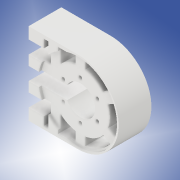
# Autodesk Inventor part: SJ001
Saved by Autodesk Inventor 2017 (Build 210142000, 142)
## iProperties
Created: 2017-06-03
Part Number: SJ001
Material: ABS Plastic
Document SubType Name: Modeling
Designer: Zach
Density: 1.06 g/cm^3
Appearance: CR White
Author: Zach
Autodesk Inventor part; units mm, degrees
ref_plane "YZ Plane" through (0, 0, 0) normal (1, 0, 0) x (0, 1, 0)
ref_plane "XZ Plane" through (0, 0, 0) normal (0, 1, 0) x (-1, 0, 0)
ref_plane "XY Plane" through (0, 0, 0) normal (0, 0, 1) x (1, 0, 0)
sketch "Sketch1" plane through (0, 0, 0) normal (0, 0, 1) x (1, 0, 0)
  circle A0 centre (0, 0) radius 62.5 construction
  line L0 (0, 62.5) -> (-75, 62.5)
  line L1 (-75, 62.5) -> (-75, -62.5)
  line L2 (-75, -62.5) -> (0, -62.5)
  arc A1 (0, -62.5) -> (0, 62.5) centre (0, 0) ccw
  dimension "d0" = 125
  dimension "d1" = 75
  dimension "d2" = 75
  constraints: 6 end point, 4 point on circle, 4 tangent, 2 centre point, 1 coincident, 1 concentric, 1 horizontal, 1 perpendicular
  measures "d0" diameter of A0
  measures "d1" distance of L0.start L0.end
  measures "d2" distance of L1.end L2.end
extrude "Extrusion1" add sketch "Sketch1" along normal blind 50
sketch "Sketch6" plane through (0, 0, 50) normal (0, 0, 1) x (1, 0, 0)
  circle A0 centre (0, 0) radius 22.5
  arc A1 (0, -62.5) -> (0, 62.5) centre (0, 0) ccw projected
  dimension "d125" = 45
  constraints: 1 centre point, 1 coincident
  measures "d125" diameter of A0
extrude "Extrusion6" cut sketch "Sketch6" against normal blind 40
sketch "Sketch7" plane through (0, 0, 50) normal (0, 0, 1) x (1, 0, 0)
  line L0 (0, 10) -> (-75, 10)
  line L1 (-75, 10) -> (-75, -10)
  line L2 (-75, -10) -> (0, -10)
  line L3 (0, -10) -> (0, 10)
  circle A0 centre (0, 0) radius 22.5 projected
  line L4 (-75, 62.5) -> (-75, -62.5) projected
  point P0 (-75, 0)
  dimension "d28" = 20
  constraints: 8 end point, 3 midpoint, 2 parallel, 1 coincident, 1 horizontal, 1 perpendicular
  measures "d28" distance of L1.end L0.end
extrude "Extrusion7" cut sketch "Sketch7" against normal blind 40 contours L3 L2 A0 L0 | A0 L2 L1 L0 picked at (-7.5, 0)
sketch "Sketch9" plane through (0, 0, 50) normal (0, 0, 1) x (1, 0, 0)
  circle A0 centre (0, 30) radius 2.5
  circle A1 centre (-25.9808, 15) radius 2.5
  circle A2 centre (-25.9808, -15) radius 2.5
  circle A3 centre (0, -30) radius 2.5
  circle A4 centre (25.9808, -15) radius 2.5
  circle A5 centre (25.9808, 15) radius 2.5
  circle A6 centre (0, 0) radius 30 construction
  dimension "d123" = 60
  dimension "d35" = 5
  dimension "d39" = 360
  constraints: 6 centre point, 2 vertical alignment, 1 coincident, 15 other
  measures "d35" diameter of A0
extrude "Extrusion9" cut sketch "Sketch9" against normal through all
sketch "Sketch10" plane through (0, 0, 50) normal (0, 0, 1) x (1, 0, 0)
  circle A0 centre (0, 0) radius 45
  arc A1 (0, -57.5) -> (0, -57.5) centre (0, 0) ccw
  line L0 (0, -57.5) -> (-75, -57.5)
  line L1 (-75, 57.5) -> (-75, -57.5)
  line L2 (0, -57.5) -> (-75, -57.5)
  line L3 (0, 57.5) -> (-75, 57.5)
  circle A2 centre (0, 0) radius 57.5 construction
  arc A3 (0, -57.5) -> (0, 57.5) centre (0, 0) ccw
  line L4 (-75, -10) -> (-75, 10)
  line L5 (0, 62.5) -> (-75, 62.5) construction
  point P0 (-75, 0)
  dimension "d111" = 115
  dimension "d43" = 90
  dimension "d114" = 90
  dimension "d124" = 5
  constraints: 10 end point, 4 point on circle, 3 centre point, 3 coincident, 2 midpoint, 2 tangent, 1 perpendicular, 1 vertical alignment, 3 other
  measures "d43" diameter of A0
  measures "d114" angle of L1 L3
  measures "d124" distance between parallel lines of L5 L3
extrude "Extrusion10" cut sketch "Sketch10" against normal blind 40
sketch "Sketch12" plane through (0, 0, 10) normal (0, 0, 1) x (1, 0, 0)
  line L0 (0, 0) -> (77.9423, -45) construction
  line L1 (0, 0) -> (90, 0) construction
  line L2 (42.1761, -15.6901) -> (57.4855, -24.529)
  line L3 (34.6761, -28.6805) -> (49.9855, -37.5194)
  arc A0 (34.6761, -28.6805) -> (42.1761, -15.6901) centre (-6.5739, 3.7955) ccw
  arc A1 (49.9877, -37.5164) -> (57.484, -24.5324) centre (-4.3593, 2.5168) ccw
  line L4 (34.6761, 28.6805) -> (49.9855, 37.5194)
  arc A2 (42.1761, 15.6901) -> (34.6761, 28.6805) centre (-6.5739, -3.7955) ccw
  line L5 (42.1761, 15.6901) -> (57.4855, 24.529)
  arc A3 (57.4855, 24.529) -> (49.9855, 37.5194) centre (-4.3593, -2.5168) ccw
  line L6 (0, 0) -> (0, -109.4234) construction
  line L7 (7.5, -44.3706) -> (7.5, -62.0484)
  line L8 (-7.5, -44.3706) -> (-7.5, -62.5)
  line L9 (0, -62.5) -> (-7.5, -62.5)
  arc A4 (-7.5, -44.3706) -> (7.5, -44.3706) centre (0, 0) ccw
  line L10 (-7.5, 44.3706) -> (-7.5, 62.5)
  line L11 (0, 62.5) -> (-7.5, 62.5)
  arc A5 (7.5, 44.3706) -> (-7.5, 44.3706) centre (0, 0) ccw
  arc A6 (-43.8748, -10) -> (-43.8748, 10) centre (0, 0) ccw projected
  arc A7 (0, -62.5) -> (0, 62.5) centre (0, 0) ccw projected
  line L12 (-75, -62.5) -> (0, -62.5) construction
  arc A8 (0, -62.5) -> (7.5, -62.0484) centre (0, 0) ccw
  line L13 (7.5, 44.3706) -> (7.5, 62.0484)
  arc A9 (7.5, 62.0484) -> (0, 62.5) centre (0, 0) ccw
  line L14 (-75, -62.5) -> (0, -62.5) projected
  line L15 (0, 62.5) -> (-75, 62.5) projected
  point P0 (54.0974, -31.2332)
  point P1 (31.1247, 32.5)
  point P2 (40, 20.6155)
  dimension "d50" = 30
  dimension "d52" = 15
  dimension "d53" = 52.5
  dimension "d54" = 67.5
  dimension "d57" = 60
  dimension "d61" = 15
  constraints: 26 end point, 24 point on circle, 8 centre point, 3 concentric, 3 point on line, 2 symmetric about line, 2 vertical, 1 equal length, 1 horizontal, 1 parallel, 14 other
  measures "d50" angle of L0 L1
  measures "d52" distance between parallel lines of L3 L2
  measures "d53" radius of A0
  measures "d54" radius of A1
  measures "d61" distance between parallel lines of L8 L7
extrude "Extrusion11" add sketch "Sketch12" along normal blind 40 contours A6 A0 | L2 A7 A1 L3 A6 | A6 L4 A3 L5 | A2 A6 | A7 A1 | A3 A7 | L7 A7 L9 L8 A4 | A5 L10 L11 A7 L13
sketch "Sketch16" plane through (0, 0, 10) normal (0, 0, 1) x (1, 0, 0)
  line L0 (-75, -62.5) -> (0, -62.5) projected
  line L1 (0, 62.5) -> (-75, 62.5) projected
  line L2 (-45, -62.5) -> (-30, -62.5)
  line L3 (-30, -62.5) -> (-30, -33.541)
  line L4 (-30, 33.541) -> (-30, 62.5)
  line L5 (-30, 62.5) -> (-45, 62.5)
  line L6 (-20.1556, -10) -> (-43.8748, -10) projected
  line L7 (-43.8748, 10) -> (-20.1556, 10) projected
  line L8 (-43.8748, 10) -> (-45, 10)
  line L9 (-43.8748, -10) -> (-45, -10)
  line L10 (-45, -10) -> (-45, -62.5)
  line L11 (-45, 62.5) -> (-45, 10)
  arc A0 (-7.5, 44.3706) -> (-43.8748, 10) centre (0, 0) ccw construction
  arc A1 (-43.8748, -10) -> (-7.5, -44.3706) centre (0, 0) ccw construction
  arc A2 (-43.8748, -10) -> (-30, -33.541) centre (0, 0) ccw
  arc A3 (-30, 33.541) -> (-43.8748, 10) centre (0, 0) ccw
  circle A4 centre (0, 0) radius 45 construction
  line L12 (-45, 10) -> (-45, -10) construction
  dimension "d127" = 15
  constraints: 18 end point, 7 point on line, 4 concentric, 4 point on circle, 3 centre point, 2 collinear, 2 vertical, 2 vertical alignment, 1 coincident, 1 perpendicular, 1 tangent
  measures "d127" distance of L2.start L2.end
extrude "Extrusion14" add sketch "Sketch16" along normal blind 40
sketch "Sketch17" plane through (0, 0, 10) normal (0, 0, 1) x (1, 0, 0)
  line L0 (-45, 10) -> (-75, 10)
  line L1 (-75, -57.5) -> (-75, 57.5) projected
  line L2 (-45, 25) -> (-75, 25)
  line L3 (-45, -10) -> (-75, -10)
  line L4 (-45, -25) -> (-75, -25)
  line L5 (-45, 25) -> (-45, 10)
  line L6 (-75, 25) -> (-75, 10)
  line L7 (-75, -10) -> (-75, -25)
  line L8 (-45, -10) -> (-45, -25)
  point P0 (0, 0)
  dimension "d39" = 360
  dimension "d72" = 15
  dimension "d73" = 15
  constraints: 16 end point, 3 point on line, 2 coincident, 2 collinear, 2 horizontal, 2 perpendicular
  measures "d72" distance between parallel lines of L0 L2
  measures "d73" distance between parallel lines of L4 L3
extrude "Extrusion15" add sketch "Sketch17" along normal blind 40
sketch "Sketch19" plane through (0, 0, 10) normal (0, 0, 1) x (1, 0, 0)
  line L0 (-75, 62.5) -> (-51.5388, 62.5)
  line L1 (-75, 25) -> (-75, 10) projected
  line L2 (-51.5388, 62.5) -> (-75, 62.5)
  line L3 (-75, 62.5) -> (-75, 45)
  line L4 (-75, 45) -> (-51.5388, 45)
  line L5 (-51.5388, 45) -> (-51.5388, 62.5)
  line L6 (-51.5388, -62.5) -> (-75, -62.5)
  line L7 (-75, 62.5) -> (-75, -62.5) projected
  line L8 (-51.5388, -62.5) -> (-75, -62.5)
  line L9 (-75, -62.5) -> (-75, -45)
  line L10 (-75, -45) -> (-51.5388, -45)
  line L11 (-51.5388, -45) -> (-51.5388, -62.5)
  point P0 (0, 0)
  point P1 (-75, -25)
  dimension "d84" = 17.5
  dimension "d85" = 17.5
  constraints: 20 end point, 4 parallel, 2 horizontal, 2 perpendicular, 2 point on line
  measures "d84" distance of L3.end L2.end
  measures "d85" distance of L8.end L9.end
extrude "Extrusion16" add sketch "Sketch19" along normal blind 40
sketch "Sketch18" plane through (-75, -62.5, 0) normal (-1, 0, 0) x (0, 0, 1)
  circle A0 centre (40, 45) radius 2.5
  circle A1 centre (20, 45) radius 2.5
  line L0 (0, 125) -> (0, 0) projected
  circle A2 centre (40, 80) radius 2.5
  circle A3 centre (20, 80) radius 2.5
  circle A4 centre (20, 116.25) radius 2.5
  circle A5 centre (20, 8.75) radius 2.5
  circle A6 centre (40, 8.75) radius 2.5
  circle A7 centre (40, 116.25) radius 2.5
  line L1 (0, 125) -> (50, 125) projected
  line L2 (10, 87.5) -> (50, 87.5) projected
  line L3 (10, 52.5) -> (50, 52.5) projected
  line L4 (0, 0) -> (50, 0) projected
  line L5 (50, 52.5) -> (50, 37.5) projected
  point P0 (0, 62.5)
  dimension "d76" = 5
  dimension "d77" = 5
  dimension "d80" = 20
  dimension "d91" = 5
  dimension "d92" = 5
  dimension "d94" = 5
  dimension "d95" = 5
  dimension "d96" = 5
  dimension "d97" = 5
  dimension "d115" = 8.75
  dimension "d116" = 7.5
  dimension "d118" = 8.75
  dimension "d129" = 7.5
  constraints: 8 centre point, 6 vertical alignment, 4 horizontal alignment
  measures "d76" diameter of A0
  measures "d77" diameter of A1
  measures "d80" distance of A1.centre A0.centre
  measures "d91" diameter of A2
  measures "d92" diameter of A3
  measures "d94" diameter of A4
  measures "d95" diameter of A5
  measures "d96" diameter of A6
  measures "d97" diameter of A7
  measures "d115" distance from line of L1 A7.centre
  measures "d116" distance from line of L2 A2.centre
  measures "d118" distance from line of L4 A6.centre
  measures "d129" distance from line of A0.centre L3
extrude "Extrusion18" cut sketch "Sketch18" against normal blind 25
sketch "Sketch22" plane through (0, 0, 50) normal (0, 0, 1) x (1, 0, 0)
  arc A0 (0, -62.5) -> (0, 62.5) centre (0, 0) ccw projected
  circle A1 centre (0, 0) radius 60
  point P0 (0, 0)
  dimension "d122" = 120
  constraints: 1 centre point, 1 coincident
  measures "d122" diameter of A1
extrude "Extrusion20" cut sketch "Sketch22" against normal blind 4.2
body "Solid1"
